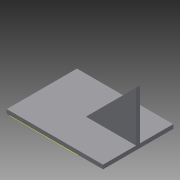
# Autodesk Inventor part: hinge_support
Saved by Autodesk Inventor 2015 SP1 (Build 190203100, 203)
## iProperties
Created: 2015-04-19
Part Number: hinge_support
Material: Ogólny
Document SubType Name: Modeling
Designer: Marcin
Density: 1 g/cm^3
Appearance: Domyślna
Author: Marcin
Autodesk Inventor part; units mm, degrees
ref_plane "YZ Plane" through (0, 0, 0) normal (1, 0, 0) x (0, 1, 0)
ref_plane "XZ Plane" through (0, 0, 0) normal (0, 1, 0) x (-1, 0, 0)
ref_plane "XY Plane" through (0, 0, 0) normal (0, 0, 1) x (1, 0, 0)
ref_plane "Płaszczyzna konstrukcyjna1" through (3.373, 0, 0) normal (0, 0, 1) x (1, 0, 0)
sketch "Szkic1" plane through (3.373, 0, 0) normal (0, 0, 1) x (1, 0, 0)
  line L0 (-18.9331, -17.5) -> (46.8447, -17.5)
  line L1 (46.8447, -17.5) -> (46.8447, 17.5)
  line L2 (46.8447, 17.5) -> (-18.9331, 17.5)
  line L3 (-18.9331, 17.5) -> (-18.9331, -17.5)
  line L4 (-3.373, 0) -> (-37.9313, 0) construction
  line L5 (46.8447, 48.9998) -> (46.8447, 17.425) construction
  arc A0 (-19.7109, 13.5) -> (-19.7109, 10.5) centre (-19.7109, 12) ccw construction
  line L6 (-19.7109, 13.5) -> (-16.7109, 13.5) construction
  arc A1 (-16.7109, 10.5) -> (-16.7109, 13.5) centre (-16.7109, 12) ccw construction
  line L7 (-16.7109, 10.5) -> (-19.7109, 10.5) construction
  line L8 (-29.2109, -13.5) -> (-32.2109, -13.5) construction
  arc A2 (-32.2109, -10.5) -> (-32.2109, -13.5) centre (-32.2109, -12) ccw construction
  line L9 (-32.2109, -10.5) -> (-29.2109, -10.5) construction
  arc A3 (-29.2109, -13.5) -> (-29.2109, -10.5) centre (-29.2109, -12) ccw construction
  circle A4 centre (-16.7109, -12) radius 1.5 construction
  circle A5 centre (-32.2109, 12) radius 1.5 construction
  line L10 (-11.7109, 6.9) -> (-34.7109, 6.9) construction
  line L11 (-11.7109, -6.9) -> (-11.7109, 6.9) construction
  line L12 (-34.7109, -6.9) -> (-11.7109, -6.9) construction
  line L13 (-15.7109, -16) -> (-34.7109, -16) construction
  line L14 (-6.2109, -9.5) -> (-15.7109, -16) construction
  line L15 (-6.2109, 9.5) -> (-6.2109, -9.5) construction
  line L16 (-15.7109, 16) -> (-6.2109, 9.5) construction
  line L17 (-34.7109, 16) -> (-15.7109, 16) construction
  line L18 (-34.7109, -6.9) -> (-34.7109, -16) projected
  line L19 (-34.7109, 16) -> (-34.7109, 6.9) projected
  dimension "d0" = 35
  constraints: 10 end point, 2 horizontal, 2 parallel, 1 collinear, 1 perpendicular, 1 other
  measures "d0" distance between parallel lines of L0 L2
extrude "Wyciągnięcie proste1" add sketch "Szkic1" along normal blind 2
sketch "Szkic2" plane through (0, 0, 0) normal (0, 1, 0) x (-1, 0, 0)
  line L0 (-50.2177, 2) -> (15.5601, 2) projected
  line L1 (-50.2177, 2) -> (-50.2177, 27)
  line L2 (-50.2177, 27) -> (-25.2177, 2)
  line L3 (-50.2177, 2) -> (-25.2177, 2)
  point P0 (0, 0)
  dimension "d3" = 25
  dimension "d4" = 25
  constraints: 6 end point, 1 point on line, 1 vertical
  measures "d3" distance of L2.end L0.start
  measures "d4" distance of L0.start L1.end
extrude "Wyciągnięcie proste2" add sketch "Szkic2" along normal mid plane 2
sketch "Szkic3" plane through (3.373, 0, 2) normal (0, 0, 1) x (1, 0, 0)
  line L0 (-18.9331, 17.5) -> (-18.9331, -17.5) projected
  line L1 (-18.9331, -17.5) -> (-10.9331, -17.5)
  line L2 (-10.9331, -17.5) -> (-10.9331, 17.5)
  line L3 (-10.9331, 17.5) -> (-18.9331, 17.5)
  line L4 (-18.9331, 17.5) -> (-18.9331, -17.5)
  point P0 (-3.373, 0)
  dimension "d7" = 8
  constraints: 8 end point, 2 parallel, 1 horizontal, 1 perpendicular
  measures "d7" distance between parallel lines of L0 L2
extrude "Wyciągnięcie proste3" cut sketch "Szkic3" against normal up to next
sketch "Szkic5" plane through (3.373, 0, 2) normal (0, 0, 1) x (1, 0, 0)
  circle A0 centre (-5.7553, 12.075) radius 1.5 projected
  arc A1 (9.7447, 10.575) -> (9.7447, 13.575) centre (9.7447, 12.075) ccw projected
  arc A2 (6.7447, 13.575) -> (6.7447, 10.575) centre (6.7447, 12.075) ccw projected
  arc A3 (-2.7553, -13.425) -> (-2.7553, -10.425) centre (-2.7553, -11.925) ccw projected
  arc A4 (-5.7553, -10.425) -> (-5.7553, -13.425) centre (-5.7553, -11.925) ccw projected
  circle A5 centre (9.7447, -11.925) radius 1.5 projected
  line L0 (-7.2553, -11.925) -> (11.2447, -11.925) construction
  line L1 (-5.7553, -13.425) -> (9.7447, -13.425)
  line L2 (9.7447, -10.425) -> (-5.7553, -10.425)
  arc A6 (-5.7553, -10.425) -> (-5.7553, -13.425) centre (-5.7553, -11.925) ccw
  arc A7 (9.7447, -13.425) -> (9.7447, -10.425) centre (9.7447, -11.925) ccw
  line L3 (-7.2553, 12.075) -> (11.2447, 12.075) construction
  line L4 (-5.7553, 10.575) -> (9.7447, 10.575)
  line L5 (9.7447, 13.575) -> (-5.7553, 13.575)
  arc A8 (-5.7553, 13.575) -> (-5.7553, 10.575) centre (-5.7553, 12.075) ccw
  arc A9 (9.7447, 10.575) -> (9.7447, 13.575) centre (9.7447, 12.075) ccw
  point P0 (-3.373, 0)
  point P1 (1.9947, -11.925)
  point P2 (1.9947, 12.075)
  constraints: 16 end point, 14 point on circle, 8 tangent, 4 centre point, 4 point on line, 2 horizontal alignment, 2 midpoint, 2 parallel, 1 horizontal, 3 other
extrude "Wyciągnięcie proste5" cut sketch "Szkic5" against normal up to next
